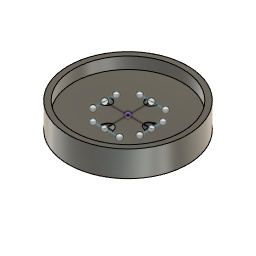
FINAL DESIGN FOR IMPINGING INJECTOR FOR HALF CIRCLE (Autodesk Fusion 360 design; units mm, degrees)
Autodesk Fusion 360 part; units mm, degrees
sketch "Sketch1" plane through (0, 0, 0) normal (0, 0, 1) x (1, 0, 0)
  circle A0 centre (0, 0) radius 50
  constraint coincident A0.centre origin
extrude "Extrude1" add sketch "Sketch1" along normal blind 20
ref_plane "WorkPlane1" through (0, 0, 10) normal (0, 0, 1) x (1, 0, 0)
sketch "Sketch2" plane through (0, 0, 10) normal (0, 0, 1) x (1, 0, 0)
  circle A0 centre (0, 0) radius 47.5
  constraint coincident A0.centre origin
extrude "Extrude2" cut sketch "Sketch2" along normal blind 10
sketch "Sketch3" plane through (0, 0, 0) normal (0, 0, 1) x (1, 0, 0)
  circle A0 centre (0, 0) radius 20
  constraint coincident A0.centre origin
extrude "Extrude3" add sketch "Sketch3" against normal blind 20
sketch "Sketch4" plane through (0, 0, -20) normal (0, 0, -1) x (1, 0, 0)
  circle A0 centre (0, 0) radius 20
shell "Shell1" thickness 1 outward yes removed faces 1 at (6.3705, -1.965, -20)
sketch "Sketch5" plane through (0, 0, 10) normal (0, 0, 1) x (1, 0, 0)
  line L0 (0, 0) -> (20, 0)
  line L1 (0, 0) -> (0, 20)
  line L2 (0, 0) -> (-20, 0)
  line L3 (0, 0) -> (0, -20)
  line L4 (-10, 20) -> (12.1822, 20)
  line L5 (-10, -20) -> (12.7429, -20)
  line L6 (-20, 10) -> (-20, -10)
  line L7 (20, 10) -> (20, -10)
  constraint coincident L0.start L1.start
  constraint horizontal L0
  constraint perpendicular L0 L1
  constraint perpendicular L1 L2
  constraint perpendicular L2 L3
  constraint perpendicular L1 L4
  constraint perpendicular L3 L5
  constraint perpendicular L2 L6
  constraint vertical L7
ref_plane "WorkPlane2" through (-20, 0, 10) normal (-0.707107, 0, 0.707107) x (0, -1, 0)
sketch "Sketch6" plane through (-20, 0, 10) normal (-0.707107, 0, 0.707107) x (0, -1, 0)
  circle A0 centre (0, 0) radius 5
  dimension "d17" = 10
  constraint coincident A0.centre origin
  measures "d17" diameter of A0
extrude "Extrude4" cut sketch "Sketch6" against normal blind 10
ref_plane "WorkPlane3" through (1.3715, -20, 10) normal (0, -0.707107, 0.707107) x (1, 0, 0)
sketch "Sketch7" plane through (0, 0, 10) normal (0, 0, 1) x (1, 0, 0)
sketch "Sketch8" plane through (1.3715, -20, 10) normal (0, -0.707107, 0.707107) x (1, 0, 0)
  circle A0 centre (0, 0) radius 5
  dimension "d21" = 10
  constraint coincident A0.centre origin
  measures "d21" diameter of A0
extrude "Extrude5" cut sketch "Sketch8" against normal blind 30
ref_plane "WorkPlane4" through (20, 0, 10) normal (0.707107, 0, 0.707107) x (0, -1, 0)
sketch "Sketch9" plane through (20, 0, 10) normal (0.707107, 0, 0.707107) x (0, -1, 0)
  circle A0 centre (0, 0) radius 5
  dimension "d25" = 10
  constraint coincident A0.centre origin
  measures "d25" diameter of A0
ref_plane "WorkPlane5" through (1.0911, 20, 10) normal (0, 0.707107, 0.707107) x (1, 0, 0)
sketch "Sketch10" plane through (1.0911, 20, 10) normal (0, 0.707107, 0.707107) x (1, 0, 0)
  circle A0 centre (0, 0) radius 5
  dimension "d27" = 10
  constraint coincident A0.centre origin
  measures "d27" diameter of A0
extrude "Extrude6" cut sketch "Sketch9" against normal blind 20
extrude "Extrude7" cut sketch "Sketch10" against normal blind 10
